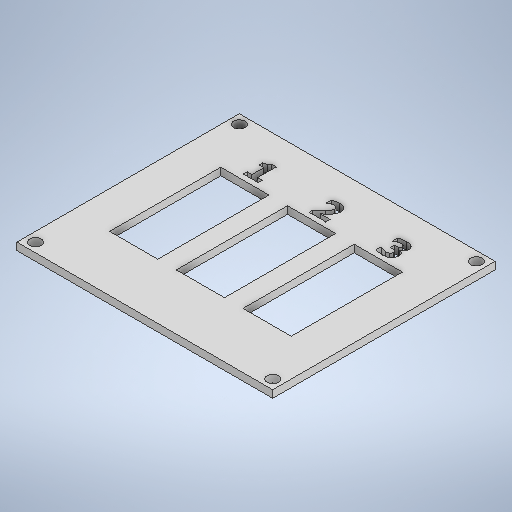
# Autodesk Inventor part: panel_switches
Saved by Autodesk Inventor 2025 (Build 290162000, 162)
## iProperties
Created: 2025-01-22
Part Number: panel_switches
Material: Generic
Document SubType Name: Modeling
Designer: danielrachi
Density: 1 g/cm^3
Appearance: Default
Author: danielrachi
Autodesk Inventor part; units mm, degrees
ref_plane "YZ Plane" through (0, 0, 0) normal (1, 0, 0) x (0, 1, 0)
ref_plane "XZ Plane" through (0, 0, 0) normal (0, 1, 0) x (-1, 0, 0)
sketch "Sketch1" plane through (0, 0, 0) normal (0, 1, 0) x (-1, 0, 0)
  line L0 (-34.5, 30) -> (34.5, 30)
  line L1 (34.5, 30) -> (34.5, -30)
  line L2 (34.5, -30) -> (-34.5, -30)
  line L3 (-34.5, -30) -> (-34.5, 30)
  line L4 (-34.5, 30) -> (34.5, -30) construction
  line L5 (34.5, 30) -> (-34.5, -30) construction
  point P0 (0, 0)
  dimension "d0" = 69
  dimension "d1" = 60
  constraints: 12 end point, 2 midpoint, 2 parallel, 1 horizontal, 1 perpendicular
  measures "d0" distance of L1.end L2.end
  measures "d1" distance of L0.end L1.end
extrude "Extrusion1" add sketch "Sketch1" along normal blind 2
sketch "Sketch2" plane through (0, 2, 0) normal (0, 1, 0) x (1, 0, 0)
  line L0 (6.5, -15) -> (-6.5, -15)
  line L1 (-6.5, -15) -> (-6.5, 15)
  line L2 (-6.5, 15) -> (6.5, 15)
  line L3 (6.5, 15) -> (6.5, -15)
  line L4 (6.5, -15) -> (-6.5, 15) construction
  line L5 (-6.5, -15) -> (6.5, 15) construction
  line L6 (-24.5, -15) -> (-11.5, -15)
  line L7 (-11.5, -15) -> (-11.5, 15)
  line L8 (-11.5, 15) -> (-24.5, 15)
  line L9 (-24.5, 15) -> (-24.5, -15)
  line L10 (-24.5, -15) -> (-11.5, 15) construction
  line L11 (-11.5, -15) -> (-24.5, 15) construction
  line L12 (-24.5, 23) -> (-11.5, 23) construction
  line L13 (-11.5, 23) -> (-11.5, 16) construction
  line L14 (-11.5, 16) -> (-24.5, 16) construction
  line L15 (-24.5, 16) -> (-24.5, 23) construction
  line L16 (-6.5, 23) -> (6.5, 23) construction
  line L17 (6.5, 23) -> (6.5, 16) construction
  line L18 (6.5, 16) -> (-6.5, 16) construction
  line L19 (-6.5, 16) -> (-6.5, 23) construction
  line L20 (11.5, -15) -> (24.5, -15)
  line L21 (24.5, -15) -> (24.5, 15)
  line L22 (24.5, 15) -> (11.5, 15)
  line L23 (11.5, 15) -> (11.5, -15)
  line L24 (11.5, -15) -> (24.5, 15) construction
  line L25 (24.5, -15) -> (11.5, 15) construction
  line L26 (11.5, 23) -> (24.5, 23) construction
  line L27 (24.5, 23) -> (24.5, 16) construction
  line L28 (24.5, 16) -> (11.5, 16) construction
  line L29 (11.5, 16) -> (11.5, 23) construction
  circle A0 centre (32, -27.5) radius 1.55
  line L30 (-34.5, -30) -> (34.5, -30) projected
  line L31 (34.5, -30) -> (34.5, 30) projected
  circle A1 centre (32, 27.5) radius 1.55
  circle A2 centre (-32, 27.5) radius 1.55
  circle A3 centre (-32, -27.5) radius 1.55
  line L32 (34.5, 30) -> (-34.5, 30) projected
  line L33 (-34.5, 30) -> (-34.5, -30) projected
  line L34 (-15.8423, 16.4426) -> (-19.871, 16.4426)
  line L35 (-19.871, 16.4426) -> (-19.871, 17.5054)
  line L36 (-19.871, 17.5054) -> (-18.5858, 17.5054)
  line L37 (-18.5858, 17.5054) -> (-18.5858, 20.7333)
  line L38 (-18.5858, 20.7333) -> (-19.871, 20.7333)
  line L39 (-19.871, 20.7333) -> (-19.871, 21.7269)
  spline S0 degree 2 poles (-19.871, 21.7269) (-19.5893, 21.7269) (-19.0307, 21.8011) (-18.8626, 21.8802) knots 0 0 0 1 2 2 2
  spline S1 degree 2 poles (-18.8626, 21.8802) (-18.6698, 21.9791) (-18.4523, 22.3103) (-18.4325, 22.5574) knots 0 0 0 1 2 2 2
  line L40 (-18.4325, 22.5574) -> (-17.0979, 22.5574)
  line L41 (-17.0979, 22.5574) -> (-17.0979, 17.5054)
  line L42 (-17.0979, 17.5054) -> (-15.8423, 17.5054)
  line L43 (-15.8423, 17.5054) -> (-15.8423, 16.4426)
  line L44 (2.4296, 16.3907) -> (-2.0539, 16.3907)
  line L45 (-2.0539, 16.3907) -> (-2.0539, 17.3843)
  spline S2 degree 2 poles (-2.0539, 17.3843) (-1.4855, 17.8391) (-0.5759, 18.6399) (-0.2348, 19.0007) knots 0 0 0 1 2 2 2
  spline S3 degree 2 poles (-0.2348, 19.0007) (0.215, 19.4703) (0.6154, 20.1871) (0.6154, 20.5628) knots 0 0 0 1 2 2 2
  spline S4 degree 2 poles (0.6154, 20.5628) (0.6154, 20.9879) (0.1063, 21.4427) (-0.3485, 21.4427) knots 0 0 0 1 2 2 2
  spline S5 degree 2 poles (-0.3485, 21.4427) (-0.5808, 21.4427) (-0.9961, 21.329) (-1.2086, 21.24) knots 0 0 0 1 2 2 2
  spline S6 degree 2 poles (-1.2086, 21.24) (-1.4162, 21.1461) (-1.7128, 20.9484) (-1.787, 20.8989) knots 0 0 0 1 2 2 2
  line L46 (-1.787, 20.8989) -> (-1.9056, 20.8989)
  line L47 (-1.9056, 20.8989) -> (-1.9056, 22.2287)
  spline S7 degree 2 poles (-1.9056, 22.2287) (-1.6486, 22.3523) (-0.5512, 22.6093) (-0.042, 22.6093) knots 0 0 0 1 2 2 2
  spline S8 degree 2 poles (-0.042, 22.6093) (1.0455, 22.6093) (2.1627, 21.6404) (2.1627, 20.7655) knots 0 0 0 1 2 2 2
  spline S9 degree 2 poles (2.1627, 20.7655) (2.1627, 20.2267) (1.6535, 19.1886) (1.0653, 18.5954) knots 0 0 0 1 2 2 2
  spline S10 degree 2 poles (1.0653, 18.5954) (0.6945, 18.2296) (-0.0025, 17.6611) (-0.1557, 17.5425) knots 0 0 0 1 2 2 2
  line L48 (-0.1557, 17.5425) -> (2.4296, 17.5425)
  line L49 (2.4296, 17.5425) -> (2.4296, 16.3907)
  spline S11 degree 2 poles (20.2764, 18.2988) (20.2764, 17.8489) (19.9452, 17.1124) (19.6239, 16.8553) knots 0 0 0 1 2 2 2
  spline S12 degree 2 poles (19.6239, 16.8553) (19.3026, 16.5983) (18.4276, 16.3215) (17.7998, 16.3215) knots 0 0 0 1 2 2 2
  spline S13 degree 2 poles (17.7998, 16.3215) (17.088, 16.3215) (16.0697, 16.5588) (15.7483, 16.7071) knots 0 0 0 1 2 2 2
  line L50 (15.7483, 16.7071) -> (15.7483, 18.0318)
  line L51 (15.7483, 18.0318) -> (15.8966, 18.0318)
  spline S14 degree 2 poles (15.8966, 18.0318) (16.2328, 17.8193) (17.1374, 17.5029) (17.5131, 17.5029) knots 0 0 0 1 2 2 2
  spline S15 degree 2 poles (17.5131, 17.5029) (17.7355, 17.5029) (18.2546, 17.582) (18.4325, 17.7105) knots 0 0 0 1 2 2 2
  spline S16 degree 2 poles (18.4325, 17.7105) (18.5709, 17.8143) (18.739, 18.1159) (18.739, 18.3878) knots 0 0 0 1 2 2 2
  spline S17 degree 2 poles (18.739, 18.3878) (18.739, 18.6596) (18.5017, 18.9513) (18.304, 19.0205) knots 0 0 0 1 2 2 2
  spline S18 degree 2 poles (18.304, 19.0205) (18.1063, 19.0897) (17.5576, 19.1045) (17.345, 19.1045) knots 0 0 0 1 2 2 2
  line L52 (17.345, 19.1045) -> (17.083, 19.1045)
  line L53 (17.083, 19.1045) -> (17.083, 20.1772)
  line L54 (17.083, 20.1772) -> (17.3252, 20.1772)
  spline S19 degree 2 poles (17.3252, 20.1772) (17.6021, 20.1772) (18.0717, 20.2267) (18.2348, 20.3008) knots 0 0 0 1 2 2 2
  spline S20 degree 2 poles (18.2348, 20.3008) (18.3979, 20.3799) (18.5808, 20.6567) (18.5808, 20.894) knots 0 0 0 1 2 2 2
  spline S21 degree 2 poles (18.5808, 20.894) (18.5808, 21.0818) (18.4078, 21.3142) (18.2842, 21.3784) knots 0 0 0 1 2 2 2
  spline S22 degree 2 poles (18.2842, 21.3784) (18.1359, 21.4526) (17.7405, 21.502) (17.6021, 21.502) knots 0 0 0 1 2 2 2
  spline S23 degree 2 poles (17.6021, 21.502) (17.3796, 21.502) (16.91, 21.3982) (16.6925, 21.3142) knots 0 0 0 1 2 2 2
  spline S24 degree 2 poles (16.6925, 21.3142) (16.5195, 21.2499) (16.1438, 21.0423) (16.0548, 20.9879) knots 0 0 0 1 2 2 2
  line L55 (16.0548, 20.9879) -> (15.9263, 20.9879)
  line L56 (15.9263, 20.9879) -> (15.9263, 22.2929)
  spline S25 degree 2 poles (15.9263, 22.2929) (16.2427, 22.4264) (17.3104, 22.6785) (17.869, 22.6785) knots 0 0 0 1 2 2 2
  spline S26 degree 2 poles (17.869, 22.6785) (18.4128, 22.6785) (19.2136, 22.4907) (19.4953, 22.3078) knots 0 0 0 1 2 2 2
  spline S27 degree 2 poles (19.4953, 22.3078) (19.8068, 22.115) (20.1182, 21.5218) (20.1182, 21.1511) knots 0 0 0 1 2 2 2
  spline S28 degree 2 poles (20.1182, 21.1511) (20.1182, 20.6271) (19.5151, 19.846) (19.0208, 19.7323) knots 0 0 0 1 2 2 2
  line L57 (19.0208, 19.7323) -> (19.0208, 19.673)
  spline S29 degree 2 poles (19.0208, 19.673) (19.2383, 19.6434) (19.6535, 19.4852) (19.8513, 19.3072) knots 0 0 0 1 2 2 2
  spline S30 degree 2 poles (19.8513, 19.3072) (20.0342, 19.149) (20.2764, 18.6448) (20.2764, 18.2988) knots 0 0 0 1 2 2 2
  point P0 (0, 0)
  point P1 (-18, 0)
  point P2 (18, 0)
  dimension "d4" = 13
  dimension "d5" = 30
  dimension "d8" = 5
  dimension "d9" = 1
  dimension "d10" = 8
  dimension "d13" = 5
  dimension "d15" = 3.1
  dimension "d16" = 2.5
  dimension "d17" = 2.5
  dimension "d18" = 2.5
  dimension "d19" = 2.5
  constraints: 36 end point, 12 collinear, 6 midpoint, 6 parallel, 4 centre point, 4 equal length, 3 equal radius, 3 horizontal, 3 perpendicular, 2 horizontal alignment, 2 vertical alignment, 6 other
  measures "d4" distance of L1.end L2.end
  measures "d5" distance of L0.end L1.end
  measures "d8" distance between parallel lines of L7 L1
  measures "d9" distance between parallel lines of L14 L8
  measures "d10" distance between parallel lines of L12 L8
  measures "d13" distance between parallel lines of L23 L3
  measures "d15" diameter of A0
  measures "d16" distance from line of A0.centre L30
  measures "d17" distance from line of A0.centre L31
  measures "d18" distance from line of A2.centre L32
  measures "d19" distance from line of A2.centre L33
extrude "Extrusion2" cut sketch "Sketch2" against normal blind 2 contours L0 L1 L2 L3 | L9 L8 L7 L6 | L23 L22 L21 L20 | A0 | A1 | A2 | A3 | L34 L35 L36 L37 L38 L39 S0 S1 L40 L41 L42 L43 | L44 L45 S2 S3 S4 S5 S6 L46 L47 S7 S8 S9 S10 L48 L49 | S11 S12 S13 L50 L51 S14 S15 S16 S17 S18 L52 L53 L54 S19 S20 S21 S22 S23 S24 L55 L56 S25 S26 S27 S28 L57 S29 S30
ref_plane "Work Plane2" through (0, 0, 30) normal (1, 0, 0) x (0, 0, -1)
equation "\"d4\" = switch_len_at_clip"
equation "\"d5\" = switch_width_at_clip"
equation "\"switch_len_at_clip\" = 13"
equation "\"switch_width_at_clip\" = 30"
equation "\"pannel_height\" = 1"
body "Solid1"
